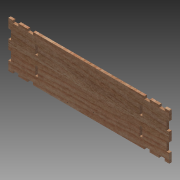
# Autodesk Inventor part: baseboard
Saved by Autodesk Inventor 2015 (Build 190159000, 159)
## iProperties
Created: 2013-12-24
Part Number: baseboard
Material: Wood (Birch)
Document SubType Name: Modeling
Designer: aoki
Density: 1 g/cm^3
Appearance: Birch - Natural Polished
Author: aoki
Autodesk Inventor part; units mm, degrees
ref_plane "YZ Plane" through (0, 0, 0) normal (1, 0, 0) x (0, 1, 0)
ref_plane "XZ Plane" through (0, 0, 0) normal (0, 1, 0) x (-1, 0, 0)
ref_plane "XY Plane" through (0, 0, 0) normal (0, 0, 1) x (1, 0, 0)
sketch "Block1" plane through (0, 0, 0) normal (0, 0, 1) x (1, 0, 0)
  line L0 (-117.6, 50.1) -> (117.6, 50.1)
  line L1 (117.6, 50.1) -> (117.6, 41.1)
  line L2 (117.6, 41.1) -> (129.4, 41.1)
  line L3 (129.4, 41.1) -> (129.4, 50.1)
  line L4 (129.4, 50.1) -> (149.6, 50.1)
  line L5 (149.6, 50.1) -> (149.6, 41.1)
  line L6 (149.6, 41.1) -> (161.4, 41.1)
  line L7 (161.4, 41.1) -> (161.4, 50.1)
  line L8 (161.4, 50.1) -> (175.1, 50.1)
  line L9 (175.1, 50.1) -> (175.1, 29.9)
  line L10 (175.1, 29.9) -> (166.1, 29.9)
  line L11 (166.1, 29.9) -> (166.1, 10.1)
  line L12 (166.1, 10.1) -> (175.1, 10.1)
  line L13 (175.1, 10.1) -> (175.1, -10.1)
  line L14 (175.1, -10.1) -> (166.1, -10.1)
  line L15 (166.1, -10.1) -> (166.1, -29.9)
  line L16 (166.1, -29.9) -> (175.1, -29.9)
  line L17 (175.1, -29.9) -> (175.1, -50.1)
  line L18 (175.1, -50.1) -> (161.4, -50.1)
  line L19 (161.4, -50.1) -> (161.4, -41.1)
  line L20 (161.4, -41.1) -> (149.6, -41.1)
  line L21 (149.6, -41.1) -> (149.6, -50.1)
  line L22 (149.6, -50.1) -> (129.4, -50.1)
  line L23 (129.4, -50.1) -> (129.4, -41.1)
  line L24 (129.4, -41.1) -> (117.6, -41.1)
  line L25 (117.6, -41.1) -> (117.6, -50.1)
  line L26 (117.6, -50.1) -> (-117.6, -50.1)
  line L27 (-117.6, -50.1) -> (-117.6, -41.1)
  line L28 (-117.6, -41.1) -> (-129.4, -41.1)
  line L29 (-129.4, -41.1) -> (-129.4, -50.1)
  line L30 (-129.4, -50.1) -> (-149.6, -50.1)
  line L31 (-149.6, -50.1) -> (-149.6, -41.1)
  line L32 (-149.6, -41.1) -> (-161.4, -41.1)
  line L33 (-161.4, -41.1) -> (-161.4, -50.1)
  line L34 (-161.4, -50.1) -> (-175.1, -50.1)
  line L35 (-175.1, -50.1) -> (-175.1, -29.9)
  line L36 (-175.1, -29.9) -> (-166.1, -29.9)
  line L37 (-166.1, -29.9) -> (-166.1, -10.1)
  line L38 (-166.1, -10.1) -> (-175.1, -10.1)
  line L39 (-175.1, -10.1) -> (-175.1, 10.1)
  line L40 (-175.1, 10.1) -> (-166.1, 10.1)
  line L41 (-166.1, 10.1) -> (-166.1, 29.9)
  line L42 (-166.1, 29.9) -> (-175.1, 29.9)
  line L43 (-175.1, 29.9) -> (-175.1, 50.1)
  line L44 (-175.1, 50.1) -> (-161.4, 50.1)
  line L45 (-161.4, 50.1) -> (-161.4, 41.1)
  line L46 (-161.4, 41.1) -> (-149.6, 41.1)
  line L47 (-149.6, 41.1) -> (-149.6, 50.1)
  line L48 (-149.6, 50.1) -> (-129.4, 50.1)
  line L49 (-129.4, 50.1) -> (-129.4, 41.1)
  line L50 (-129.4, 41.1) -> (-117.6, 41.1)
  line L51 (-117.6, 41.1) -> (-117.6, 50.1)
  line L52 (-103.9, 30.1) -> (-103.9, 9.9)
  line L53 (-103.9, 9.9) -> (-113.1, 9.9)
  line L54 (-113.1, 9.9) -> (-113.1, 30.1)
  line L55 (-113.1, 30.1) -> (-103.9, 30.1)
  line L56 (-103.9, -9.9) -> (-113.1, -9.9)
  line L57 (-113.1, -9.9) -> (-113.1, -30.1)
  line L58 (-113.1, -30.1) -> (-103.9, -30.1)
  line L59 (-103.9, -30.1) -> (-103.9, -9.9)
  line L60 (113.1, 30.1) -> (113.1, 9.9)
  line L61 (113.1, 9.9) -> (103.9, 9.9)
  line L62 (103.9, 9.9) -> (103.9, 30.1)
  line L63 (103.9, 30.1) -> (113.1, 30.1)
  line L64 (113.1, -9.9) -> (103.9, -9.9)
  line L65 (103.9, -9.9) -> (103.9, -30.1)
  line L66 (103.9, -30.1) -> (113.1, -30.1)
  line L67 (113.1, -30.1) -> (113.1, -9.9)
  point P0 (0, 0)
sketch "Block2" plane through (0, 0, 0) normal (0, 0, 1) x (1, 0, 0)
  line L0 (-117.7, 50.2) -> (117.7, 50.2)
  line L1 (117.7, 50.2) -> (117.7, 41.2)
  line L2 (117.7, 41.2) -> (129.3, 41.2)
  line L3 (129.3, 41.2) -> (129.3, 50.2)
  line L4 (129.3, 50.2) -> (149.7, 50.2)
  line L5 (149.7, 50.2) -> (149.7, 41.2)
  line L6 (149.7, 41.2) -> (161.3, 41.2)
  line L7 (161.3, 41.2) -> (161.3, 50.2)
  line L8 (161.3, 50.2) -> (175.2, 50.2)
  line L9 (175.2, 50.2) -> (175.2, 29.8)
  line L10 (175.2, 29.8) -> (166.2, 29.8)
  line L11 (166.2, 29.8) -> (166.2, 10.2)
  line L12 (166.2, 10.2) -> (175.2, 10.2)
  line L13 (175.2, 10.2) -> (175.2, -10.2)
  line L14 (175.2, -10.2) -> (166.2, -10.2)
  line L15 (166.2, -10.2) -> (166.2, -29.8)
  line L16 (166.2, -29.8) -> (175.2, -29.8)
  line L17 (175.2, -29.8) -> (175.2, -50.2)
  line L18 (175.2, -50.2) -> (161.3, -50.2)
  line L19 (161.3, -50.2) -> (161.3, -41.2)
  line L20 (161.3, -41.2) -> (149.7, -41.2)
  line L21 (149.7, -41.2) -> (149.7, -50.2)
  line L22 (149.7, -50.2) -> (129.3, -50.2)
  line L23 (129.3, -50.2) -> (129.3, -41.2)
  line L24 (129.3, -41.2) -> (117.7, -41.2)
  line L25 (117.7, -41.2) -> (117.7, -50.2)
  line L26 (117.7, -50.2) -> (-117.7, -50.2)
  line L27 (-117.7, -50.2) -> (-117.7, -41.2)
  line L28 (-117.7, -41.2) -> (-129.3, -41.2)
  line L29 (-129.3, -41.2) -> (-129.3, -50.2)
  line L30 (-129.3, -50.2) -> (-149.7, -50.2)
  line L31 (-149.7, -50.2) -> (-149.7, -41.2)
  line L32 (-149.7, -41.2) -> (-161.3, -41.2)
  line L33 (-161.3, -41.2) -> (-161.3, -50.2)
  line L34 (-161.3, -50.2) -> (-175.2, -50.2)
  line L35 (-175.2, -50.2) -> (-175.2, -29.8)
  line L36 (-175.2, -29.8) -> (-166.2, -29.8)
  line L37 (-166.2, -29.8) -> (-166.2, -10.2)
  line L38 (-166.2, -10.2) -> (-175.2, -10.2)
  line L39 (-175.2, -10.2) -> (-175.2, 10.2)
  line L40 (-175.2, 10.2) -> (-166.2, 10.2)
  line L41 (-166.2, 10.2) -> (-166.2, 29.8)
  line L42 (-166.2, 29.8) -> (-175.2, 29.8)
  line L43 (-175.2, 29.8) -> (-175.2, 50.2)
  line L44 (-175.2, 50.2) -> (-161.3, 50.2)
  line L45 (-161.3, 50.2) -> (-161.3, 41.2)
  line L46 (-161.3, 41.2) -> (-149.7, 41.2)
  line L47 (-149.7, 41.2) -> (-149.7, 50.2)
  line L48 (-149.7, 50.2) -> (-129.3, 50.2)
  line L49 (-129.3, 50.2) -> (-129.3, 41.2)
  line L50 (-129.3, 41.2) -> (-117.7, 41.2)
  line L51 (-117.7, 41.2) -> (-117.7, 50.2)
  line L52 (-103.8, 30.2) -> (-103.8, 9.8)
  line L53 (-103.8, 9.8) -> (-113.2, 9.8)
  line L54 (-113.2, 9.8) -> (-113.2, 30.2)
  line L55 (-113.2, 30.2) -> (-103.8, 30.2)
  line L56 (-103.8, -9.8) -> (-113.2, -9.8)
  line L57 (-113.2, -9.8) -> (-113.2, -30.2)
  line L58 (-113.2, -30.2) -> (-103.8, -30.2)
  line L59 (-103.8, -30.2) -> (-103.8, -9.8)
  line L60 (113.2, 30.2) -> (113.2, 9.8)
  line L61 (113.2, 9.8) -> (103.8, 9.8)
  line L62 (103.8, 9.8) -> (103.8, 30.2)
  line L63 (103.8, 30.2) -> (113.2, 30.2)
  line L64 (113.2, -9.8) -> (103.8, -9.8)
  line L65 (103.8, -9.8) -> (103.8, -30.2)
  line L66 (103.8, -30.2) -> (113.2, -30.2)
  line L67 (113.2, -30.2) -> (113.2, -9.8)
  point P0 (0, 0)
sketch "Block3" plane through (0, 0, 0) normal (0, 0, 1) x (1, 0, 0)
  line L0 (-117.6, 50.1) -> (117.6, 50.1)
  line L1 (117.6, 50.1) -> (117.6, 41.1)
  line L2 (117.6, 41.1) -> (129.4, 41.1)
  line L3 (129.4, 41.1) -> (129.4, 50.1)
  line L4 (129.4, 50.1) -> (149.6, 50.1)
  line L5 (149.6, 50.1) -> (149.6, 41.1)
  line L6 (149.6, 41.1) -> (161.4, 41.1)
  line L7 (161.4, 41.1) -> (161.4, 50.1)
  line L8 (161.4, 50.1) -> (175.1, 50.1)
  line L9 (175.1, 50.1) -> (175.1, 29.9)
  line L10 (175.1, 29.9) -> (166.1, 29.9)
  line L11 (166.1, 29.9) -> (166.1, 10.1)
  line L12 (166.1, 10.1) -> (175.1, 10.1)
  line L13 (175.1, 10.1) -> (175.1, -10.1)
  line L14 (175.1, -10.1) -> (166.1, -10.1)
  line L15 (166.1, -10.1) -> (166.1, -29.9)
  line L16 (166.1, -29.9) -> (175.1, -29.9)
  line L17 (175.1, -29.9) -> (175.1, -50.1)
  line L18 (175.1, -50.1) -> (161.4, -50.1)
  line L19 (161.4, -50.1) -> (161.4, -41.1)
  line L20 (161.4, -41.1) -> (149.6, -41.1)
  line L21 (149.6, -41.1) -> (149.6, -50.1)
  line L22 (149.6, -50.1) -> (129.4, -50.1)
  line L23 (129.4, -50.1) -> (129.4, -41.1)
  line L24 (129.4, -41.1) -> (117.6, -41.1)
  line L25 (117.6, -41.1) -> (117.6, -50.1)
  line L26 (117.6, -50.1) -> (-117.6, -50.1)
  line L27 (-117.6, -50.1) -> (-117.6, -41.1)
  line L28 (-117.6, -41.1) -> (-129.4, -41.1)
  line L29 (-129.4, -41.1) -> (-129.4, -50.1)
  line L30 (-129.4, -50.1) -> (-149.6, -50.1)
  line L31 (-149.6, -50.1) -> (-149.6, -41.1)
  line L32 (-149.6, -41.1) -> (-161.4, -41.1)
  line L33 (-161.4, -41.1) -> (-161.4, -50.1)
  line L34 (-161.4, -50.1) -> (-175.1, -50.1)
  line L35 (-175.1, -50.1) -> (-175.1, -29.9)
  line L36 (-175.1, -29.9) -> (-166.1, -29.9)
  line L37 (-166.1, -29.9) -> (-166.1, -10.1)
  line L38 (-166.1, -10.1) -> (-175.1, -10.1)
  line L39 (-175.1, -10.1) -> (-175.1, 10.1)
  line L40 (-175.1, 10.1) -> (-166.1, 10.1)
  line L41 (-166.1, 10.1) -> (-166.1, 29.9)
  line L42 (-166.1, 29.9) -> (-175.1, 29.9)
  line L43 (-175.1, 29.9) -> (-175.1, 50.1)
  line L44 (-175.1, 50.1) -> (-161.4, 50.1)
  line L45 (-161.4, 50.1) -> (-161.4, 41.1)
  line L46 (-161.4, 41.1) -> (-149.6, 41.1)
  line L47 (-149.6, 41.1) -> (-149.6, 50.1)
  line L48 (-149.6, 50.1) -> (-129.4, 50.1)
  line L49 (-129.4, 50.1) -> (-129.4, 41.1)
  line L50 (-129.4, 41.1) -> (-117.6, 41.1)
  line L51 (-117.6, 41.1) -> (-117.6, 50.1)
  line L52 (-103.9, 30.1) -> (-103.9, 9.9)
  line L53 (-103.9, 9.9) -> (-113.1, 9.9)
  line L54 (-113.1, 9.9) -> (-113.1, 30.1)
  line L55 (-113.1, 30.1) -> (-103.9, 30.1)
  line L56 (-103.9, -9.9) -> (-113.1, -9.9)
  line L57 (-113.1, -9.9) -> (-113.1, -30.1)
  line L58 (-113.1, -30.1) -> (-103.9, -30.1)
  line L59 (-103.9, -30.1) -> (-103.9, -9.9)
  line L60 (113.1, 30.1) -> (113.1, 9.9)
  line L61 (113.1, 9.9) -> (103.9, 9.9)
  line L62 (103.9, 9.9) -> (103.9, 30.1)
  line L63 (103.9, 30.1) -> (113.1, 30.1)
  line L64 (113.1, -9.9) -> (103.9, -9.9)
  line L65 (103.9, -9.9) -> (103.9, -30.1)
  line L66 (103.9, -30.1) -> (113.1, -30.1)
  line L67 (113.1, -30.1) -> (113.1, -9.9)
  point P0 (0, 0)
sketch "Block4" plane through (0, 0, 0) normal (0, 0, 1) x (1, 0, 0)
  line L0 (-121.08, 50.08) -> (121.08, 50.08)
  line L1 (121.08, 50.08) -> (121.08, 44.58)
  line L2 (121.08, 44.58) -> (132.92, 44.58)
  line L3 (132.92, 44.58) -> (132.92, 50.08)
  line L4 (132.92, 50.08) -> (153.08, 50.08)
  line L5 (153.08, 50.08) -> (153.08, 44.58)
  line L6 (153.08, 44.58) -> (164.92, 44.58)
  line L7 (164.92, 44.58) -> (164.92, 50.08)
  line L8 (164.92, 50.08) -> (175.08, 50.08)
  line L9 (175.08, 50.08) -> (175.08, 29.92)
  line L10 (175.08, 29.92) -> (169.58, 29.92)
  line L11 (169.58, 29.92) -> (169.58, 10.08)
  line L12 (169.58, 10.08) -> (175.08, 10.08)
  line L13 (175.08, 10.08) -> (175.08, -10.08)
  line L14 (175.08, -10.08) -> (169.58, -10.08)
  line L15 (169.58, -10.08) -> (169.58, -29.92)
  line L16 (169.58, -29.92) -> (175.08, -29.92)
  line L17 (175.08, -29.92) -> (175.08, -50.08)
  line L18 (175.08, -50.08) -> (164.92, -50.08)
  line L19 (164.92, -50.08) -> (164.92, -44.58)
  line L20 (164.92, -44.58) -> (153.08, -44.58)
  line L21 (153.08, -44.58) -> (153.08, -50.08)
  line L22 (153.08, -50.08) -> (132.92, -50.08)
  line L23 (132.92, -50.08) -> (132.92, -44.58)
  line L24 (132.92, -44.58) -> (121.08, -44.58)
  line L25 (121.08, -44.58) -> (121.08, -50.08)
  line L26 (121.08, -50.08) -> (-121.08, -50.08)
  line L27 (-121.08, -50.08) -> (-121.08, -44.58)
  line L28 (-121.08, -44.58) -> (-132.92, -44.58)
  line L29 (-132.92, -44.58) -> (-132.92, -50.08)
  line L30 (-132.92, -50.08) -> (-153.08, -50.08)
  line L31 (-153.08, -50.08) -> (-153.08, -44.58)
  line L32 (-153.08, -44.58) -> (-164.92, -44.58)
  line L33 (-164.92, -44.58) -> (-164.92, -50.08)
  line L34 (-164.92, -50.08) -> (-175.08, -50.08)
  line L35 (-175.08, -50.08) -> (-175.08, -29.92)
  line L36 (-175.08, -29.92) -> (-169.58, -29.92)
  line L37 (-169.58, -29.92) -> (-169.58, -10.08)
  line L38 (-169.58, -10.08) -> (-175.08, -10.08)
  line L39 (-175.08, -10.08) -> (-175.08, 10.08)
  line L40 (-175.08, 10.08) -> (-169.58, 10.08)
  line L41 (-169.58, 10.08) -> (-169.58, 29.92)
  line L42 (-169.58, 29.92) -> (-175.08, 29.92)
  line L43 (-175.08, 29.92) -> (-175.08, 50.08)
  line L44 (-175.08, 50.08) -> (-164.92, 50.08)
  line L45 (-164.92, 50.08) -> (-164.92, 44.58)
  line L46 (-164.92, 44.58) -> (-153.08, 44.58)
  line L47 (-153.08, 44.58) -> (-153.08, 50.08)
  line L48 (-153.08, 50.08) -> (-132.92, 50.08)
  line L49 (-132.92, 50.08) -> (-132.92, 44.58)
  line L50 (-132.92, 44.58) -> (-121.08, 44.58)
  line L51 (-121.08, 44.58) -> (-121.08, 50.08)
  line L52 (-110.92, 30.08) -> (-110.92, 9.92)
  line L53 (-110.92, 9.92) -> (-116.58, 9.92)
  line L54 (-116.58, 9.92) -> (-116.58, 30.08)
  line L55 (-116.58, 30.08) -> (-110.92, 30.08)
  line L56 (-110.92, -9.92) -> (-116.58, -9.92)
  line L57 (-116.58, -9.92) -> (-116.58, -30.08)
  line L58 (-116.58, -30.08) -> (-110.92, -30.08)
  line L59 (-110.92, -30.08) -> (-110.92, -9.92)
  line L60 (116.58, 30.08) -> (116.58, 9.92)
  line L61 (116.58, 9.92) -> (110.92, 9.92)
  line L62 (110.92, 9.92) -> (110.92, 30.08)
  line L63 (110.92, 30.08) -> (116.58, 30.08)
  line L64 (116.58, -9.92) -> (110.92, -9.92)
  line L65 (110.92, -9.92) -> (110.92, -30.08)
  line L66 (110.92, -30.08) -> (116.58, -30.08)
  line L67 (116.58, -30.08) -> (116.58, -9.92)
  point P0 (0, 0)
sketch "Sketch1" plane through (0, 0, 0) normal (0, 1, 0) x (-1, 0, 0)
  line L0 (175, -50) -> (-175, -50)
  line L1 (-175, -50) -> (-175, 50)
  line L2 (-175, 50) -> (175, 50)
  line L3 (175, 50) -> (175, -50)
  line L4 (175, -50) -> (-175, 50) construction
  line L5 (-175, -50) -> (175, 50) construction
  line L6 (0, 0) -> (0, 75.8521)
  dimension "d0" = 350
  dimension "d1" = 100
  constraints: 14 end point, 3 parallel, 2 midpoint, 1 horizontal, 1 perpendicular
  measures "d0" distance of L1.end L2.end
  measures "d1" distance of L0.end L1.end
extrude "Extrusion1" add sketch "Sketch1" along normal blind 5.5
sketch "Sketch6" plane through (0, 5.5, 0) normal (0, 1, 0) x (1, 0, 0)
  line L0 (175, 50) -> (-175, 50) projected
  line L1 (-175, 50) -> (-175, -50) projected
  line L2 (175, -50) -> (175, 50) projected
  line L3 (-116.5, 30) -> (-111, 30)
  line L4 (-111, 30) -> (-111, 10)
  line L5 (-111, 10) -> (-116.5, 10)
  line L6 (-116.5, 10) -> (-116.5, 30)
  line L7 (-175, 30) -> (-169.5, 30)
  line L8 (-169.5, 30) -> (-169.5, 10)
  line L9 (-169.5, 10) -> (-175, 10)
  line L10 (-175, 10) -> (-175, 30)
  line L11 (111, 30) -> (116.5, 30)
  line L12 (116.5, 30) -> (116.5, 10)
  line L13 (116.5, 10) -> (111, 10)
  line L14 (111, 10) -> (111, 30)
  line L15 (169.5, 30) -> (175, 30)
  line L16 (175, 30) -> (175, 10)
  line L17 (175, 10) -> (169.5, 10)
  line L18 (169.5, 10) -> (169.5, 30)
  line L19 (-321.0918, 0) -> (700.8506, 0) projected
  line L20 (0, 73.9124) -> (0, -70.7687) projected
  line L21 (-116.5, -30) -> (-111, -30)
  line L22 (-111, -30) -> (-111, -10)
  line L23 (-111, -10) -> (-116.5, -10)
  line L24 (-116.5, -10) -> (-116.5, -30)
  line L25 (-175, -30) -> (-169.5, -30)
  line L26 (-169.5, -30) -> (-169.5, -10)
  line L27 (-169.5, -10) -> (-175, -10)
  line L28 (-175, -10) -> (-175, -30)
  line L29 (111, -30) -> (116.5, -30)
  line L30 (116.5, -30) -> (116.5, -10)
  line L31 (116.5, -10) -> (111, -10)
  line L32 (111, -10) -> (111, -30)
  line L33 (169.5, -30) -> (175, -30)
  line L34 (175, -30) -> (175, -10)
  line L35 (175, -10) -> (169.5, -10)
  line L36 (169.5, -10) -> (169.5, -30)
  point P0 (0, 0)
  dimension "d31" = 20
  dimension "d32" = 20
  dimension "d33" = 20
  dimension "d34" = 20
  dimension "d35" = 20
  dimension "d36" = 20
  dimension "d37" = 20
  dimension "d38" = 20
  dimension "d39" = 5.5
  dimension "d40" = 5.5
  dimension "d41" = 5.5
  dimension "d42" = 5.5
  dimension "d43" = 53
  dimension "d44" = 53
  constraints: 64 end point, 16 symmetric about line, 8 parallel, 4 horizontal, 4 perpendicular, 2 collinear
  measures "d31" distance between parallel lines of L0 L3
  measures "d32" distance between parallel lines of L7 L0
  measures "d33" distance between parallel lines of L0 L11
  measures "d34" distance between parallel lines of L0 L15
  measures "d35" distance of L3.end L4.end
  measures "d36" distance of L7.end L8.end
  measures "d37" distance of L11.end L12.end
  measures "d38" distance of L15.end L16.end
  measures "d39" distance of L8.end L9.end
  measures "d40" distance of L4.end L5.end
  measures "d41" distance of L12.end L13.end
  measures "d42" distance of L16.end L17.end
  measures "d43" distance between parallel lines of L8 L6
  measures "d44" distance between parallel lines of L18 L12
extrude "Extrusion2" cut sketch "Sketch6" against normal through all contours L2 L33 L36 L35 | L27 L26 L25 L1 | L2 L17 L18 L15 | L7 L8 L9 L1 | L3 L4 L5 L6 | L11 L12 L13 L14 | L24 L23 L22 L21 | L32 L31 L30 L29
sketch "Sketch8" plane through (0, 0, 0) normal (0, -1, 0) x (1, 0, 0)
  line L0 (-175, -50) -> (175, -50) projected
  line L1 (111, 30) -> (116.5, 30) projected
  line L2 (-175, 59.2811) -> (-175, -60.1862)
  line L3 (-111, 61.9963) -> (-111, -60.1862)
  line L4 (-143, 61.9963) -> (-143, -69.2367)
  line L5 (-321.0918, 0) -> (700.8506, 0) projected
  line L6 (-153, -50) -> (-165, -50)
  line L7 (-165, -50) -> (-165, -44.5)
  line L8 (-165, -44.5) -> (-153, -44.5)
  line L9 (-153, -44.5) -> (-153, -50)
  line L10 (-133, -50) -> (-121, -50)
  line L11 (-121, -50) -> (-121, -44.5)
  line L12 (-121, -44.5) -> (-133, -44.5)
  line L13 (-133, -44.5) -> (-133, -50)
  line L14 (-153, 50) -> (-165, 50)
  line L15 (-165, 50) -> (-165, 44.5)
  line L16 (-165, 44.5) -> (-153, 44.5)
  line L17 (-153, 44.5) -> (-153, 50)
  line L18 (-121, 44.5) -> (-133, 44.5)
  line L19 (-133, 44.5) -> (-133, 50)
  line L20 (-121, 50) -> (-121, 44.5)
  line L21 (-133, 50) -> (-121, 50)
  line L22 (175, -10) -> (175, 10) projected
  line L23 (0, 69.8052) -> (0, -77.7744)
  line L24 (153, -50) -> (165, -50)
  line L25 (165, -50) -> (165, -44.5)
  line L26 (165, -44.5) -> (153, -44.5)
  line L27 (153, -44.5) -> (153, -50)
  line L28 (121, -44.5) -> (133, -44.5)
  line L29 (133, -44.5) -> (133, -50)
  line L30 (121, -50) -> (121, -44.5)
  line L31 (133, -50) -> (121, -50)
  line L32 (121, 50) -> (121, 44.5)
  line L33 (121, 44.5) -> (133, 44.5)
  line L34 (133, 50) -> (121, 50)
  line L35 (133, 44.5) -> (133, 50)
  line L36 (153, 44.5) -> (153, 50)
  line L37 (165, 44.5) -> (153, 44.5)
  line L38 (153, 50) -> (165, 50)
  line L39 (165, 50) -> (165, 44.5)
  line L40 (-175, 50) -> (-175, 30) projected
  point P0 (117.5, -50)
  point P1 (0, 0)
  dimension "d54" = 12
  dimension "d55" = 20
  dimension "d58" = 5.5
  dimension "d61" = 64
  constraints: 72 end point, 28 symmetric about line, 5 parallel, 2 perpendicular, 1 collinear, 1 horizontal, 1 point on line, 1 other
  measures "d54" distance of L7.end L8.end
  measures "d55" distance between parallel lines of L13 L9
  measures "d58" distance of L11.start L12.start
  measures "d61" distance between parallel lines of L3 L2
extrude "Extrusion5" cut sketch "Sketch8" against normal through all contours L27 L26 L25 L0 | L30 L28 L29 L0 | L7 L8 L9 L0 | L13 L12 L11 L0 | L17 L16 L15 L14 | L18 L19 L21 L20 | L34 L35 L33 L32 | L36 L38 L39 L37
equation "\"d0\" = Base_length"
equation "\"d2\" = Wt"
equation "\"d39\" = Wt"
equation "\"d40\" = Wt"
equation "\"d41\" = Wt"
equation "\"d42\" = Wt"
equation "\"d58\" = Wt"
equation "\"Base_length\" = 350"
equation "\"Wt\" = 5.5"
body "Solid1"
